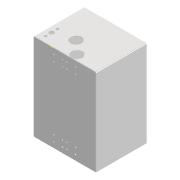
# Autodesk Inventor part: Part75
Saved by Autodesk Inventor 2020.5 (Build 245400000, 400)
## iProperties
Created: 2022-11-22
Part Number: Part75
Material: 一般
Document SubType Name: Sheet Metal
Designer: Administrator
Density: 1 g/cm^3
Appearance: 既定
Sheet Metal Rule: Default_mm
Author: Administrator
Autodesk Inventor part; units mm, degrees
ref_plane "YZ Plane" through (0, 0, 0) normal (1, 0, 0) x (0, 1, 0)
ref_plane "XZ Plane" through (0, 0, 0) normal (0, 1, 0) x (-1, 0, 0)
ref_plane "XY Plane" through (0, 0, 0) normal (0, 0, 1) x (1, 0, 0)
sketch "スケッチ1" plane through (0, 0, 0) normal (0, 0, 1) x (1, 0, 0)
  line L0 (28.45, -63.6) -> (28.45, -61) projected
  line L1 (28.45, -61) -> (31.5, -61) projected
  line L2 (31.5, -20.4) -> (31.5, -61) projected
  line L3 (2, -20.4) -> (31.5, -20.4) projected
  line L4 (2, -20.4) -> (2, -61) projected
  line L5 (2, -61) -> (5.05, -61) projected
  line L6 (5.05, -61) -> (5.05, -63.6) projected
  line L7 (28.45, -63.6) -> (5.05, -63.6) projected
  circle A0 centre (28, -50) radius 1.35 projected
  circle A1 centre (5.5, -34) radius 1.35 projected
  circle A2 centre (5.5, -50) radius 1.35 projected
  circle A3 centre (28, -34) radius 1.35 projected
  line L8 (38.55, -63.6) -> (61.95, -63.6) projected
  line L9 (61.95, -61) -> (61.95, -63.6) projected
  line L10 (65, -61) -> (61.95, -61) projected
  line L11 (65, -20.4) -> (65, -61) projected
  line L12 (65, -20.4) -> (35.5, -20.4) projected
  line L13 (35.5, -20.4) -> (35.5, -61) projected
  line L14 (38.55, -61) -> (35.5, -61) projected
  line L15 (38.55, -63.6) -> (38.55, -61) projected
  circle A4 centre (61.5, -34) radius 1.35 projected
  circle A5 centre (39, -50) radius 1.35 projected
  circle A6 centre (61.5, -50) radius 1.35 projected
  circle A7 centre (39, -34) radius 1.35 projected
  line L16 (28.45, -179.4) -> (28.45, -182) projected
  line L17 (28.45, -179.4) -> (5.05, -179.4) projected
  line L18 (5.05, -182) -> (5.05, -179.4) projected
  line L19 (2, -182) -> (5.05, -182) projected
  line L20 (2, -222.6) -> (2, -182) projected
  line L21 (2, -222.6) -> (31.5, -222.6) projected
  line L22 (31.5, -222.6) -> (31.5, -182) projected
  line L23 (28.45, -182) -> (31.5, -182) projected
  circle A8 centre (28, -193) radius 1.35 projected
  circle A9 centre (5.5, -209) radius 1.35 projected
  circle A10 centre (5.5, -193) radius 1.35 projected
  circle A11 centre (28, -209) radius 1.35 projected
  line L24 (38.55, -179.4) -> (61.95, -179.4) projected
  line L25 (38.55, -179.4) -> (38.55, -182) projected
  line L26 (38.55, -182) -> (35.5, -182) projected
  line L27 (35.5, -222.6) -> (35.5, -182) projected
  line L28 (65, -222.6) -> (35.5, -222.6) projected
  line L29 (65, -222.6) -> (65, -182) projected
  line L30 (65, -182) -> (61.95, -182) projected
  line L31 (61.95, -182) -> (61.95, -179.4) projected
  circle A12 centre (61.5, -209) radius 1.35 projected
  circle A13 centre (39, -193) radius 1.35 projected
  circle A14 centre (61.5, -193) radius 1.35 projected
  circle A15 centre (39, -209) radius 1.35 projected
  line L32 (-44.591, -20) -> (-44.591, -31) projected
  line L33 (-44.591, -223) -> (-44.591, -212) projected
  line L34 (111.591, -223) -> (111.591, -213) projected
  line L35 (111.591, -20) -> (111.591, -30) projected
  line L36 (31.5, -20.4) -> (-46.5, -20.4)
  line L37 (35.5, -20.4) -> (113.5, -20.4)
  line L38 (-46.4989, -223.01) -> (-46.5, -20.4)
  line L39 (113.5, -20.4) -> (113.4989, -223.01)
  circle A16 centre (61.5, -34) radius 1.6
  circle A17 centre (61.5, -50) radius 1.6
  circle A18 centre (39, -34) radius 1.6
  circle A19 centre (39, -50) radius 1.6
  circle A20 centre (28, -34) radius 1.6
  circle A21 centre (28, -50) radius 1.6
  circle A22 centre (5.5, -50) radius 1.6
  circle A23 centre (5.5, -34) radius 1.6
  circle A24 centre (61.5, -193) radius 1.6
  circle A25 centre (61.5, -209) radius 1.6
  circle A26 centre (39, -193) radius 1.6
  circle A27 centre (39, -209) radius 1.6
  circle A28 centre (28, -193) radius 1.6
  circle A29 centre (28, -209) radius 1.6
  circle A30 centre (5.5, -209) radius 1.6
  circle A31 centre (5.5, -193) radius 1.6
  line L40 (23.0262, -20.4) -> (42.9971, -20.4)
  line L41 (-46.4989, -223.01) -> (113.4989, -223.01)
  point P0 (0, 0)
  point P1 (65, -20.4)
  point P2 (35.5, -20.4)
  point P3 (23.0262, -20.4)
  point P4 (2, -20.4)
  dimension "d0" = 78
  dimension "d3" = 78
  dimension "d4" = 78
  dimension "d5" = 78
  dimension "d6" = 3.2
  dimension "d7" = 3.2
  dimension "d8" = 3.2
  dimension "d9" = 3.2
  dimension "d10" = 3.2
  dimension "d11" = 3.2
  dimension "d12" = 3.2
  dimension "d13" = 3.2
  dimension "d14" = 3.2
  dimension "d15" = 3.2
  dimension "d16" = 3.2
  dimension "d17" = 3.2
  dimension "d18" = 3.2
  dimension "d19" = 3.2
  dimension "d20" = 3.2
  dimension "d21" = 3.2
  constraints: 16 centre point, 16 coincident, 12 end point, 3 horizontal, 2 point on line
  measures "d0" distance of L2.start L36.end
  measures "d3" distance of L12.end L37.end
  measures "d4" distance of L27.start L39.end
  measures "d5" distance of L21.end L38.start
  measures "d6" diameter of A16
  measures "d7" diameter of A17
  measures "d8" diameter of A18
  measures "d9" diameter of A19
  measures "d10" diameter of A20
  measures "d11" diameter of A21
  measures "d12" diameter of A22
  measures "d13" diameter of A23
  measures "d14" diameter of A24
  measures "d15" diameter of A25
  measures "d16" diameter of A26
  measures "d17" diameter of A27
  measures "d18" diameter of A28
  measures "d19" diameter of A29
  measures "d20" diameter of A30
  measures "d21" diameter of A31
sketch "スケッチ2" plane through (0, 0, 0) normal (0, 1, 0) x (-1, 0, 0)
  point P0 (0, 0)
extrude "押し出し1" add sketch "スケッチ1" along normal blind 1 contours L7 L6 L5 L4 L3 L2 L1 L0 | L0 L1 L2 L40 L13 L14 L15 L8 L9 L10 L11 L37 L39 L41 L38 L36 L4 L5 L6 L7 | L12 L11 L10 L9 L8 L15 L14 L13 | L16 L23 L22 L21 L20 L19 L18 L17 | L24 L31 L30 L29 L28 L27 L26 L25
sketch "スケッチ3" plane through (114.4989, -223.01, -1) normal (1, -0.0000053, 0) x (0.0000053, 1, 0)
  line L0 (202.61, 0) -> (0, 0)
  line L1 (0, 0) -> (0, -128)
  line L2 (0, -128) -> (202.61, -128)
  line L3 (202.61, -128) -> (202.61, 0)
  constraints: 6 end point, 1 horizontal, 1 perpendicular, 1 vertical
edge flange "フランジ1" height 130 angle 90 thickness 1 bend radius 1 thickness toward (1, -0.0000053, 0) relief straight relief width 1 relief depth 0.5 corner gap 1 corner form 0 edges at (113.4995, -121.705, 0) (-46.4995, -121.705, 0) wall of the first edge with corners at (114.5, -20.4, -1) (114.4989, -223.01, -1) (114.4989, -223.01, -129) (114.5, -20.4, -129)
bend "曲げ1"
corner "コーナー1"
sketch "スケッチ6" plane through (113.5, -19.4, -1) normal (0, 1, 0) x (-1, 0, 0)
  line L0 (160, 0) -> (0, 0)
  line L1 (0, 0) -> (0, -78)
  line L2 (0, -78) -> (160, -78)
  line L3 (160, -78) -> (160, 0)
  constraints: 6 end point, 1 horizontal, 1 perpendicular, 1 vertical
edge flange "フランジ3" height 80 angle 90 thickness 1 bend radius 1 thickness toward (0, 1, 0) relief straight relief width 1 relief depth 0.5 corner gap 1 corner form 0 edges at (33.5, -20.4, 0) (33.5, -223.01, 0) wall of the first edge with corners at (-46.5, -19.4, -1) (113.5, -19.4, -1) (113.5, -19.4, -79) (-46.5, -19.4, -79)
bend "曲げ3"
corner "コーナー3"
ref_plane "作業平面1" through (-47.4989, -223.01, -128) normal (-1, -0.0000053, 0) x (0, 0, 1)
sketch "スケッチ8" plane through (-47.4989, -223.01, -128) normal (-1, -0.0000053, 0) x (0, 0, 1)
  line L0 (69.5, 180.01) -> (69.5, 30.01) projected
  line L1 (69.5, 30.01) -> (109.5, 30.01) projected
  line L2 (109.5, 180.01) -> (109.5, 30.01) projected
  line L3 (69.5, 180.01) -> (109.5, 180.01) projected
  line L4 (0, 202.61) -> (127, 202.61) projected
  line L5 (127, 0) -> (0, 0) projected
  ellipse E0 centre (98, 9.01) end of major axis (109, 9.01) minor radius 0.0001 projected
  line L6 (62, 15) -> (117, 15)
  line L7 (117, 15) -> (117, 187.61)
  line L8 (117, 187.61) -> (62, 187.61)
  line L9 (62, 187.61) -> (62, 15)
  line L10 (127, 1) -> (127, 201.61) projected
  point P0 (128, 223.0098)
  dimension "d72" = 55
  dimension "d74" = 202.61
  dimension "d75" = 15
  dimension "d76" = 10
  dimension "d85" = 15
  constraints: 8 end point, 2 parallel, 1 horizontal, 1 perpendicular
  measures "d72" distance of L8.end L7.end
  measures "d74" distance between parallel lines of L4 L5
  measures "d75" distance between parallel lines of L6 L5
  measures "d76" distance between parallel lines of L10 L7
  measures "d85" distance between parallel lines of L4 L8
extrude "押し出し3" cut sketch "スケッチ8" against normal through all both and the other way through all contours L3 L2 L1 L0 | L9 L8 L7 L6
sketch "スケッチ9" plane through (-46.5, -18.4, -1) normal (0, 1, 0) x (1, 0, 0)
  circle A0 centre (13.909, 13.5) radius 2.5 projected
  circle A1 centre (13.909, 44.5) radius 2.5 projected
  circle A2 centre (13.909, 29) radius 11 projected
  line L0 (0.909, 13.8013) -> (0.909, 44.1987) projected
  arc A3 (0.909, 13.8013) -> (26.909, 13.8013) centre (13.909, 29) ccw projected
  line L1 (26.909, 44.1987) -> (26.909, 13.8013) projected
  arc A4 (26.909, 44.1987) -> (0.909, 44.1987) centre (13.909, 29) ccw projected
  circle A5 centre (13.909, 29) radius 4.5 projected
  circle A6 centre (62.25, 43.75) radius 13 projected
  circle A7 centre (95.75, 12.75) radius 12.8 projected
  circle A8 centre (144.091, 13.5) radius 2.5 projected
  circle A9 centre (144.091, 44.5) radius 2.5 projected
  circle A10 centre (144.091, 29) radius 11 projected
  line L2 (157.091, 13.8013) -> (157.091, 44.1987) projected
  arc A11 (157.091, 44.1987) -> (131.091, 44.1987) centre (144.091, 29) ccw projected
  line L3 (131.091, 44.1987) -> (131.091, 13.8013) projected
  arc A12 (131.091, 13.8013) -> (157.091, 13.8013) centre (144.091, 29) ccw projected
  circle A13 centre (62.25, 43.75) radius 15
  circle A14 centre (95.75, 12.75) radius 15
  circle A15 centre (13.909, 29) radius 6
  circle A16 centre (144.091, 29) radius 6
  line L4 (95.75, 12.75) -> (95.75, -2.25)
  line L5 (95.75, 12.75) -> (80.75, 12.75)
  line L6 (159.9989, 0) -> (0.0011, 0) projected
  line L7 (80.75, 0) -> (80.75, 12.75)
  line L8 (95.75, 12.75) -> (110.75, 12.75)
  line L9 (110.75, 0) -> (110.75, 12.75)
  line L10 (80.75, 0) -> (110.75, 0)
  line L11 (80.75, 12.75) -> (110.75, 12.75)
  line L12 (110.75, 12.75) -> (110.75, 27.75)
  line L13 (110.75, 27.75) -> (80.75, 27.75)
  line L14 (80.75, 27.75) -> (80.75, 12.75)
  point P0 (46.5, -1)
  point P1 (95.75, 27.75)
  dimension "d79" = 30
  dimension "d80" = 30
  dimension "d81" = 12
  dimension "d82" = 12
  dimension "d90" = 30
  constraints: 20 end point, 4 centre point, 4 coincident, 3 perpendicular, 3 point on circle, 3 point on line, 2 horizontal, 2 parallel, 2 tangent, 1 collinear, 1 vertical
  measures "d79" diameter of A13
  measures "d80" diameter of A14
  measures "d81" diameter of A15
  measures "d82" diameter of A16
  measures "d90" distance of L13.end L12.end
extrude "押し出し4" cut sketch "スケッチ9" against normal through all contours A0 | A1 | A5 | A6 | L8 L5 A7 | L8 A14 L6 A7 | A7 L6 L4 L8 | A7 L5 A14 L8 | L5 L4 L6 A7 | A7 L6 A14 L5 | L9 L6 A14 | A14 L13 L12 | L14 L13 A14 | A14 L6 L7 | A8 | A9 | A13 | A15 | A16
sketch "スケッチ10" plane through (0, 0, 1) normal (0, 0, 1) x (1, 0, 0)
  line L0 (34.25, -18.4) -> (64.25, -18.4) projected
  line L1 (34.25, -18.4) -> (64.25, -18.4)
  line L2 (64.25, -18.4) -> (64.25, -23.4)
  line L3 (64.25, -23.4) -> (34.25, -23.4)
  line L4 (34.25, -23.4) -> (34.25, -18.4)
  line L5 (64.25, -225.01) -> (34.25, -225.01) projected
  line L6 (64.25, -225.01) -> (34.25, -225.01) projected
  line L7 (34.25, -225.01) -> (64.25, -225.01)
  line L8 (64.25, -225.01) -> (64.25, -220.01)
  line L9 (64.25, -220.01) -> (34.25, -220.01)
  line L10 (34.25, -220.01) -> (34.25, -225.01)
  point P0 (0, 0)
  dimension "d94" = 5
  dimension "d95" = 5
  constraints: 16 end point, 4 parallel, 2 horizontal, 2 perpendicular
  measures "d94" distance of L1.end L2.end
  measures "d95" distance of L8.end L7.end
extrude "押し出し5" cut sketch "スケッチ10" against normal blind 10
fillet "フィレット1" radius 2 4 edges at (34.25, -18.9, -28.75) (64.25, -18.9, -28.75) (34.25, -224.51, -28.75) (64.25, -224.51, -28.75)
fillet "フィレット2" radius 2 8 edges at (114.999, -208.0092, -66) (114.999, -208.0092, -11) (114.9999, -35.3991, -11) (114.9999, -35.3991, -66) (-47.9999, -35.4, -11) (-47.999, -208.01, -66) (-47.999, -208.01, -11) (-47.9999, -35.4, -66)
fillet "フィレット3" radius 2 4 edges at (64.25, -220.01, 0.5) (34.25, -220.01, 0.5) (34.25, -23.4, 0.5) (64.25, -23.4, 0.5)
equation "\"d24\" = Thickness"
equation "\"d25\" = BendReliefWidth"
equation "\"d26\" = BendReliefDepth"
equation "\"d27\" = MinimumRemnant"
equation "\"d28\" = TransitionRadius"
equation "\"d31\" = BendRadius"
equation "\"d32\" = CornerReliefSize"
equation "\"d33\" = GapSize"
equation "\"d34\" = JacobiRadiusSize"
equation "\"d52\" = BendReliefWidth"
equation "\"d53\" = BendReliefDepth"
equation "\"d54\" = MinimumRemnant"
equation "\"d55\" = TransitionRadius"
equation "\"d58\" = BendRadius"
equation "\"d59\" = CornerReliefSize"
equation "\"d60\" = GapSize"
equation "\"d61\" = JacobiRadiusSize"
equation "\"BendRadius\" = Thickness"
equation "\"BendReliefWidth\" = Thickness"
equation "\"BendReliefDepth\" = 0.5 * Thickness"
equation "\"CornerReliefSize\" = 4 * Thickness"
equation "\"MinimumRemnant\" = 2 * Thickness"
equation "\"TransitionRadius\" = BendRadius"
equation "\"JacobiRadiusSize\" = BendRadius"
equation "\"GapSize\" = Thickness"
equation "\"Thickness\" = 1"
